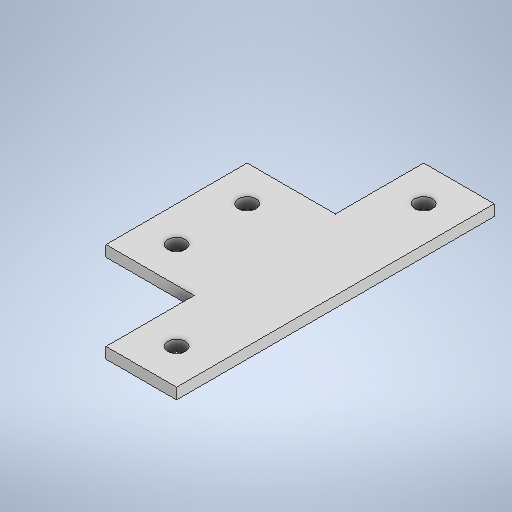
# Autodesk Inventor part: 2020DoubleT
Saved by Autodesk Inventor 2025.1 (Build 291241000, 241)
## iProperties
Created: 2025-12-08
Part Number: 2020DoubleT
Material: Generic
Document SubType Name: Modeling
Designer: Juxin
Density: 1 g/cm^3
Appearance: Default
Author: Juxin
Autodesk Inventor part; units mm, degrees
ref_plane "YZ Plane" through (0, 0, 0) normal (1, 0, 0) x (0, 1, 0)
ref_plane "XZ Plane" through (0, 0, 0) normal (0, 1, 0) x (-1, 0, 0)
ref_plane "XY Plane" through (0, 0, 0) normal (0, 0, 1) x (1, 0, 0)
sketch "Sketch1" plane through (0, 0, 0) normal (0, 1, 0) x (-1, 0, 0)
  line L0 (0, 0) -> (25.4, 0)
  line L1 (25.4, 0) -> (25.4, -40.64)
  line L2 (25.4, -40.64) -> (0, -40.64)
  line L3 (0, -40.64) -> (0, 0)
  line L4 (25.4, 0) -> (15.24, 0)
  line L5 (15.24, 0) -> (15.24, -10.16)
  line L6 (25.4, -40.64) -> (15.24, -40.64)
  line L7 (15.24, -40.64) -> (15.24, -30.48)
  circle A0 centre (15.24, -10.16) radius 2.54
  circle A1 centre (15.24, -30.48) radius 2.54
  line L8 (0, 0) -> (0, 25.4)
  line L9 (0, 0) -> (25.4, 0) construction
  line L10 (0, 25.4) -> (-20.32, 25.4)
  line L11 (-20.32, 25.4) -> (-20.32, -66.04)
  line L12 (-20.32, -66.04) -> (0, -66.04)
  line L13 (0, -66.04) -> (0, -40.64)
  line L14 (-10.16, 25.4) -> (-10.16, 15.24)
  line L15 (-10.16, 25.4) -> (0, 25.4) construction
  line L16 (-10.16, -66.04) -> (-10.16, -55.88)
  line L17 (-10.16, -66.04) -> (0, -66.04) construction
  circle A2 centre (-10.16, 15.24) radius 2.54
  circle A3 centre (-10.16, -55.88) radius 2.54
  dimension "d0" = 25.4
  dimension "d1" = 40.64
  dimension "d2" = 10.16
  dimension "d3" = 10.16
  dimension "d4" = 90
  dimension "d5" = 10.16
  dimension "d6" = 10.16
  dimension "d7" = 90
  dimension "d8" = 5.08
  dimension "d9" = 5.08
  dimension "d10" = 25.4
  dimension "d11" = 90
  dimension "d12" = 20.32
  dimension "d13" = 91.44
  dimension "d14" = 90
  dimension "d15" = 20.32
  dimension "d16" = 90
  dimension "d17" = 10.16
  dimension "d18" = 90
  dimension "d19" = 10.16
  dimension "d20" = 90
  dimension "d21" = 5.08
  dimension "d22" = 5.08
  constraints: 36 end point, 9 perpendicular, 4 centre point, 4 coincident, 4 horizontal, 3 vertical, 2 midpoint, 2 parallel, 2 point on line
  measures "d0" distance of L1.end L2.end
  measures "d1" distance of L0.end L1.end
  measures "d2" distance of L0.end L4.end
  measures "d3" distance of L4.end L5.end
  measures "d4" angle of L5 L4
  measures "d5" distance of L1.end L6.end
  measures "d6" distance of L6.end L7.end
  measures "d7" angle of L6 L7
  measures "d8" diameter of A0
  measures "d9" diameter of A1
  measures "d10" distance of L0.start L8.end
  measures "d11" angle of L9 L8
  measures "d12" distance of L8.end L10.end
  measures "d13" distance of L10.end L11.end
  measures "d14" angle of L11 L10
  measures "d15" distance of L11.end L12.end
  measures "d16" angle of L12 L11
  measures "d17" distance of L14.start L14.end
  measures "d18" angle of L14 L15
  measures "d19" distance of L16.start L16.end
  measures "d20" angle of L17 L16
  measures "d21" diameter of A2
  measures "d22" diameter of A3
extrude "Extrusion1" add sketch "Sketch1" along normal blind 3.175
body "Solid1"
